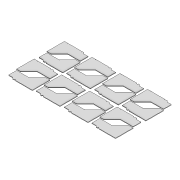
# Autodesk Inventor part: Contour_SDCard_multiple
Saved by Autodesk Inventor 2022 (Build 260153000, 153)
## iProperties
Created: 2023-04-19
Part Number: Contour_SDCard_multiple
Material: Generisch
Document SubType Name: Modeling
Designer: diederichbenedict
Density: 1 g/cm^3
Appearance: Vorgabe
Author: diederichbenedict
Autodesk Inventor part; units mm, degrees
(part 1 of 2)
ref_plane "YZ Plane" through (0, 0, 0) normal (1, 0, 0) x (0, 1, 0)
ref_plane "XZ Plane" through (0, 0, 0) normal (0, 1, 0) x (-1, 0, 0)
ref_plane "XY Plane" through (0, 0, 0) normal (0, 0, 1) x (1, 0, 0)
sketch "Skizze1" plane through (0, 0, 0) normal (0, 1, 0) x (-1, 0, 0)
  line L0 (9.6766, 36.5124) -> (7.9266, 36.5124)
  line L1 (34.6032, 1.527) -> (34.6032, 10.9706)
  line L2 (101.255, 38.0416) -> (101.255, 47.4852)
  line L3 (24.9386, 68.4228) -> (29.9386, 68.4228)
  line L4 (39.5032, 38.027) -> (34.5032, 38.027)
  line L5 (119.867, 33.452) -> (120.617, 32.702)
  line L6 (124.767, 68.452) -> (129.767, 68.452)
  line L7 (106.355, 1.5416) -> (101.355, 1.5416)
  line L8 (31.3402, 36.5124) -> (31.3402, 57.5178)
  line L9 (4.9526, 48.9174) -> (15.011, 58.9758)
  line L10 (104.781, 48.9466) -> (114.839, 59.005)
  line L11 (109.505, 36.5416) -> (107.755, 36.5416)
  line L12 (15.111, 22.4758) -> (30.0386, 22.4758)
  line L13 (77.5282, 0.777) -> (76.5282, 0.777)
  line L14 (54.7652, 69.1874) -> (54.7652, 69.9374)
  line L15 (121.517, 69.202) -> (121.517, 69.952)
  line L16 (131.168, 57.547) -> (126.241, 57.547)
  line L17 (53.0152, 69.9374) -> (53.7652, 69.1874)
  line L18 (64.5168, 21.0324) -> (59.5892, 21.0324)
  line L19 (39.6032, 1.527) -> (34.6032, 1.527)
  line L20 (78.1782, 36.527) -> (77.4282, 37.277)
  line L21 (87.5402, 32.6874) -> (88.5402, 32.6874)
  line L22 (31.3402, 57.5178) -> (26.4126, 57.5178)
  line L23 (44.5032, 36.527) -> (43.7532, 37.277)
  line L24 (53.7652, 69.1874) -> (54.7652, 69.1874)
  line L25 (126.241, 57.547) -> (116.182, 47.4886)
  line L26 (116.282, 10.9886) -> (101.355, 10.9886)
  line L27 (90.1902, 69.9374) -> (91.6902, 68.4374)
  line L28 (101.355, 1.5416) -> (101.355, 10.9852)
  line L29 (58.0152, 68.4374) -> (63.0152, 68.4374)
  line L30 (78.2782, 0.027) -> (98.1918, 0.027)
  line L31 (71.7042, 48.932) -> (81.7626, 58.9904)
  line L32 (121.617, 32.702) -> (121.617, 33.452)
  line L33 (49.5308, 10.974) -> (34.6032, 10.974)
  line L34 (88.5402, 33.4374) -> (90.2902, 33.4374)
  line L35 (31.4402, 21.0178) -> (26.5126, 21.0178)
  line L36 (90.2902, 33.4374) -> (91.7902, 31.9374)
  line L37 (111.355, 0.0416) -> (110.605, 0.7916)
  line L38 (76.4282, 37.277) -> (76.4282, 36.527)
  line L39 (9.6766, 37.2624) -> (9.6766, 36.5124)
  line L40 (86.6902, 69.9374) -> (66.7766, 69.9374)
  line L41 (111.255, 36.5416) -> (110.505, 37.2916)
  line L42 (5.0526, 12.4174) -> (15.111, 22.4758)
  line L43 (6.5266, 1.5124) -> (1.5266, 1.5124)
  line L44 (44.6032, 0.027) -> (64.5168, 0.027)
  line L45 (110.505, 37.2916) -> (109.505, 37.2916)
  line L46 (120.517, 69.202) -> (121.517, 69.202)
  line L47 (87.4402, 69.1874) -> (88.4402, 69.1874)
  line L48 (16.4542, 10.9594) -> (1.5266, 10.9594)
  line L49 (41.1032, 0.027) -> (39.6032, 1.527)
  line L50 (74.7782, 0.027) -> (73.2782, 1.527)
  line L51 (54.7652, 69.9374) -> (56.5152, 69.9374)
  line L52 (54.8652, 32.6874) -> (54.8652, 33.4374)
  line L53 (98.1918, 21.0324) -> (93.2642, 21.0324)
  line L54 (98.0918, 36.527) -> (98.0918, 57.5324)
  line L55 (129.767, 68.452) -> (129.767, 59.0084)
  line L56 (6.4266, 38.0124) -> (1.4266, 38.0124)
  line L57 (15.011, 58.9758) -> (29.9386, 58.9758)
  line L58 (1.5266, 1.5124) -> (1.5266, 10.956)
  line L59 (64.5168, 0.027) -> (64.5168, 21.0324)
  line L60 (0.025, 69.9228) -> (0.025, 48.9174)
  line L61 (21.7886, 33.4228) -> (23.5386, 33.4228)
  line L62 (64.4168, 36.527) -> (64.4168, 57.5324)
  line L63 (126.341, 21.047) -> (116.282, 10.9886)
  line L64 (66.8766, 12.432) -> (71.8042, 12.432)
  line L65 (30.0386, 31.9228) -> (30.0386, 22.4792)
  line L66 (119.767, 69.952) -> (120.517, 69.202)
  line L67 (114.939, 22.505) -> (129.867, 22.505)
  line L68 (68.1782, 38.027) -> (68.1782, 47.4706)
  line L69 (11.4266, 36.5124) -> (10.6766, 37.2624)
  line L70 (9.7766, 0.0124) -> (8.0266, 0.0124)
  line L71 (114.839, 59.005) -> (129.767, 59.005)
  line L72 (99.9532, 33.452) -> (99.9532, 12.4466)
  line L73 (11.5266, 0.0124) -> (31.4402, 0.0124)
  line L74 (71.8042, 12.432) -> (81.8626, 22.4904)
  line L75 (91.7902, 31.9374) -> (96.7902, 31.9374)
  line L76 (29.9386, 68.4228) -> (29.9386, 58.9792)
  line L77 (99.8532, 69.952) -> (99.8532, 48.9466)
  line L78 (119.767, 69.952) -> (99.8532, 69.952)
  line L79 (31.4402, 0.0124) -> (31.4402, 21.0178)
  line L80 (93.2642, 21.0324) -> (83.2058, 10.974)
  line L81 (91.6902, 68.4374) -> (96.6902, 68.4374)
  line L82 (23.4386, 69.9228) -> (24.9386, 68.4228)
  line L83 (25.0386, 31.9228) -> (30.0386, 31.9228)
  line L84 (42.7532, 37.277) -> (42.7532, 36.527)
  line L85 (8.0266, 0.0124) -> (6.5266, 1.5124)
  line L86 (66.8766, 33.4374) -> (66.8766, 12.432)
  line L87 (76.5282, 0.027) -> (74.7782, 0.027)
  line L88 (42.7532, 36.527) -> (41.0032, 36.527)
  line L89 (26.5126, 21.0178) -> (16.4542, 10.9594)
  line L90 (96.6902, 68.4374) -> (96.6902, 58.9938)
  line L91 (59.4892, 57.5324) -> (49.4308, 47.474)
  line L92 (49.4308, 47.474) -> (34.5032, 47.474)
  line L93 (20.0386, 33.4228) -> (20.7886, 32.6728)
  line L94 (26.4126, 57.5178) -> (16.3542, 47.4594)
  line L95 (109.505, 37.2916) -> (109.505, 36.5416)
  line L96 (20.6886, 69.1728) -> (21.6886, 69.1728)
  line L97 (120.617, 32.702) -> (121.617, 32.702)
  line L98 (107.755, 36.5416) -> (106.255, 38.0416)
  line L99 (123.267, 69.952) -> (124.767, 68.452)
  line L100 (86.6902, 69.9374) -> (87.4402, 69.1874)
  line L101 (48.1876, 22.4904) -> (63.1152, 22.4904)
  line L102 (21.6886, 69.9228) -> (23.4386, 69.9228)
  line L103 (56.6152, 33.4374) -> (58.1152, 31.9374)
  line L104 (1.4266, 38.0124) -> (1.4266, 47.456)
  line L105 (53.1152, 33.4374) -> (53.8652, 32.6874)
  line L106 (83.2058, 10.974) -> (68.2782, 10.974)
  line L107 (129.867, 31.952) -> (129.867, 22.5084)
  line L108 (93.1642, 57.5324) -> (83.1058, 47.474)
  line L109 (11.4266, 36.5124) -> (31.3402, 36.5124)
  line L110 (53.1152, 33.4374) -> (33.2016, 33.4374)
  line L111 (23.5386, 33.4228) -> (25.0386, 31.9228)
  line L112 (81.8626, 22.4904) -> (96.7902, 22.4904)
  line L113 (33.2016, 33.4374) -> (33.2016, 12.432)
  line L114 (42.8532, 0.777) -> (42.8532, 0.027)
  line L115 (73.2782, 1.527) -> (68.2782, 1.527)
  line L116 (20.7886, 32.6728) -> (21.7886, 32.6728)
  line L117 (73.1782, 38.027) -> (68.1782, 38.027)
  line L118 (11.5266, 0.0124) -> (10.7766, 0.7624)
  line L119 (86.7902, 33.4374) -> (87.5402, 32.6874)
  line L120 (16.3542, 47.4594) -> (1.4266, 47.4594)
  line L121 (86.7902, 33.4374) -> (66.8766, 33.4374)
  line L122 (44.6032, 0.027) -> (43.8532, 0.777)
  line L123 (43.8532, 0.777) -> (42.8532, 0.777)
  line L124 (38.0292, 48.932) -> (48.0876, 58.9904)
  line L125 (96.7902, 31.9374) -> (96.7902, 22.4938)
  line L126 (21.6886, 69.1728) -> (21.6886, 69.9228)
  line L127 (104.881, 12.4466) -> (114.939, 22.505)
  line L128 (131.268, 0.0416) -> (131.268, 21.047)
  line L129 (131.268, 21.047) -> (126.341, 21.047)
  line L130 (98.1918, 0.027) -> (98.1918, 21.0324)
  line L131 (88.4402, 69.9374) -> (90.1902, 69.9374)
  line L132 (38.1292, 12.432) -> (48.1876, 22.4904)
  line L133 (88.4402, 69.1874) -> (88.4402, 69.9374)
  line L134 (124.867, 31.952) -> (129.867, 31.952)
  line L135 (33.1016, 69.9374) -> (33.1016, 48.932)
  line L136 (10.7766, 0.7624) -> (9.7766, 0.7624)
  line L137 (43.7532, 37.277) -> (42.7532, 37.277)
  line L138 (10.6766, 37.2624) -> (9.6766, 37.2624)
  line L139 (121.517, 69.952) -> (123.267, 69.952)
  line L140 (33.1016, 48.932) -> (38.0292, 48.932)
  line L141 (81.7626, 58.9904) -> (96.6902, 58.9904)
  line L142 (76.4282, 36.527) -> (74.6782, 36.527)
  line L143 (119.867, 33.452) -> (99.9532, 33.452)
  line L144 (99.9532, 12.4466) -> (104.881, 12.4466)
  line L145 (64.4168, 57.5324) -> (59.4892, 57.5324)
  line L146 (66.7766, 48.932) -> (71.7042, 48.932)
  line L147 (110.605, 0.7916) -> (109.605, 0.7916)
  line L148 (33.2016, 12.432) -> (38.1292, 12.432)
  line L149 (78.1782, 36.527) -> (98.0918, 36.527)
  line L150 (56.5152, 69.9374) -> (58.0152, 68.4374)
  line L151 (34.5032, 38.027) -> (34.5032, 47.4706)
  line L152 (48.0876, 58.9904) -> (63.0152, 58.9904)
  line L153 (7.9266, 36.5124) -> (6.4266, 38.0124)
  line L154 (121.617, 33.452) -> (123.367, 33.452)
  line L155 (63.0152, 68.4374) -> (63.0152, 58.9938)
  line L156 (0.025, 48.9174) -> (4.9526, 48.9174)
  line L157 (99.8532, 48.9466) -> (104.781, 48.9466)
  line L158 (74.6782, 36.527) -> (73.1782, 38.027)
  line L159 (109.605, 0.0416) -> (107.855, 0.0416)
  line L160 (98.0918, 57.5324) -> (93.1642, 57.5324)
  line L161 (116.182, 47.4886) -> (101.255, 47.4886)
  line L162 (42.8532, 0.027) -> (41.1032, 0.027)
  line L163 (53.8652, 32.6874) -> (54.8652, 32.6874)
  line L164 (123.367, 33.452) -> (124.867, 31.952)
  line L165 (63.1152, 31.9374) -> (63.1152, 22.4938)
  line L166 (44.5032, 36.527) -> (64.4168, 36.527)
  line L167 (0.125, 33.4228) -> (0.125, 12.4174)
  line L168 (76.5282, 0.777) -> (76.5282, 0.027)
  line L169 (111.255, 36.5416) -> (131.168, 36.5416)
  line L170 (19.9386, 69.9228) -> (20.6886, 69.1728)
  line L171 (106.255, 38.0416) -> (101.255, 38.0416)
  line L172 (66.7766, 69.9374) -> (66.7766, 48.932)
  line L173 (109.605, 0.7916) -> (109.605, 0.0416)
  line L174 (21.7886, 32.6728) -> (21.7886, 33.4228)
  line L175 (20.0386, 33.4228) -> (0.125, 33.4228)
  line L176 (107.855, 0.0416) -> (106.355, 1.5416)
  line L177 (131.168, 36.5416) -> (131.168, 57.547)
  line L178 (53.0152, 69.9374) -> (33.1016, 69.9374)
  line L179 (59.5892, 21.0324) -> (49.5308, 10.974)
  line L180 (78.2782, 0.027) -> (77.5282, 0.777)
  line L181 (19.9386, 69.9228) -> (0.025, 69.9228)
  line L182 (58.1152, 31.9374) -> (63.1152, 31.9374)
  line L183 (41.0032, 36.527) -> (39.5032, 38.027)
  line L184 (88.5402, 32.6874) -> (88.5402, 33.4374)
  line L185 (54.8652, 33.4374) -> (56.6152, 33.4374)
  line L186 (83.1058, 47.474) -> (68.1782, 47.474)
  line L187 (9.7766, 0.7624) -> (9.7766, 0.0124)
  line L188 (111.355, 0.0416) -> (131.268, 0.0416)
  line L189 (68.2782, 1.527) -> (68.2782, 10.9706)
  line L190 (0.125, 12.4174) -> (5.0526, 12.4174)
  line L191 (77.4282, 37.277) -> (76.4282, 37.277)
  line L192 (93.9699, 35.8046) -> (93.6365, 36.2808)
  line L193 (93.3984, 35.8046) -> (93.3984, 36.8046)
  line L194 (93.3984, 36.8046) -> (93.7794, 36.8046)
  line L195 (93.7794, 36.8046) -> (93.8746, 36.757)
  line L196 (93.8746, 36.757) -> (93.9222, 36.7094)
  line L197 (93.9222, 36.7094) -> (93.9699, 36.6141)
  line L198 (93.9699, 36.6141) -> (93.9699, 36.4713)
  line L199 (93.9699, 36.4713) -> (93.9222, 36.376)
  line L200 (93.9222, 36.376) -> (93.8746, 36.3284)
  line L201 (93.8746, 36.3284) -> (93.7794, 36.2808)
  line L202 (93.7794, 36.2808) -> (93.3984, 36.2808)
  line L203 (94.3984, 36.3284) -> (94.7318, 36.3284)
  line L204 (94.8746, 35.8046) -> (94.3984, 35.8046)
  line L205 (94.3984, 35.8046) -> (94.3984, 36.8046)
  line L206 (94.3984, 36.8046) -> (94.8746, 36.8046)
  line L207 (95.6365, 36.3284) -> (95.3032, 36.3284)
  line L208 (95.3032, 35.8046) -> (95.3032, 36.8046)
  line L209 (95.3032, 36.8046) -> (95.7794, 36.8046)
  line L210 (96.3032, 36.8046) -> (96.3032, 36.5665)
  line L211 (96.0651, 36.6618) -> (96.3032, 36.5665)
  line L212 (96.3032, 36.5665) -> (96.5413, 36.6618)
  line L213 (96.1603, 36.376) -> (96.3032, 36.5665)
  line L214 (96.3032, 36.5665) -> (96.4461, 36.376)
  line L215 (97.0651, 36.8046) -> (97.0651, 36.5665)
  line L216 (96.827, 36.6618) -> (97.0651, 36.5665)
  line L217 (97.0651, 36.5665) -> (97.3032, 36.6618)
  line L218 (96.9222, 36.376) -> (97.0651, 36.5665)
  line L219 (97.0651, 36.5665) -> (97.208, 36.376)
  line L220 (34.5569, 69.925) -> (34.2235, 70.4012)
  line L221 (33.9854, 69.925) -> (33.9854, 70.925)
  line L222 (33.9854, 70.925) -> (34.3664, 70.925)
  line L223 (34.3664, 70.925) -> (34.4616, 70.8774)
  line L224 (34.4616, 70.8774) -> (34.5092, 70.8298)
  line L225 (34.5092, 70.8298) -> (34.5569, 70.7345)
  line L226 (34.5569, 70.7345) -> (34.5569, 70.5917)
  line L227 (34.5569, 70.5917) -> (34.5092, 70.4964)
  line L228 (34.5092, 70.4964) -> (34.4616, 70.4488)
  line L229 (34.4616, 70.4488) -> (34.3664, 70.4012)
  line L230 (34.3664, 70.4012) -> (33.9854, 70.4012)
  line L231 (34.9854, 70.4488) -> (35.3188, 70.4488)
  line L232 (35.4616, 69.925) -> (34.9854, 69.925)
  line L233 (34.9854, 69.925) -> (34.9854, 70.925)
  line L234 (34.9854, 70.925) -> (35.4616, 70.925)
  line L235 (36.2235, 70.4488) -> (35.8902, 70.4488)
  line L236 (35.8902, 69.925) -> (35.8902, 70.925)
  line L237 (35.8902, 70.925) -> (36.3664, 70.925)
  line L238 (36.8902, 70.925) -> (36.8902, 70.6869)
  line L239 (36.6521, 70.7822) -> (36.8902, 70.6869)
  line L240 (36.8902, 70.6869) -> (37.1283, 70.7822)
  line L241 (36.7473, 70.4964) -> (36.8902, 70.6869)
  line L242 (36.8902, 70.6869) -> (37.0331, 70.4964)
  line L243 (37.6521, 70.925) -> (37.6521, 70.6869)
  line L244 (37.414, 70.7822) -> (37.6521, 70.6869)
  line L245 (37.6521, 70.6869) -> (37.8902, 70.7822)
  line L246 (37.5092, 70.4964) -> (37.6521, 70.6869)
  line L247 (37.6521, 70.6869) -> (37.795, 70.4964)
  line L248 (68.3319, 33.425) -> (67.9985, 33.9012)
  line L249 (67.7604, 33.425) -> (67.7604, 34.425)
  line L250 (67.7604, 34.425) -> (68.1414, 34.425)
  line L251 (68.1414, 34.425) -> (68.2366, 34.3774)
  line L252 (68.2366, 34.3774) -> (68.2842, 34.3298)
  line L253 (68.2842, 34.3298) -> (68.3319, 34.2345)
  line L254 (68.3319, 34.2345) -> (68.3319, 34.0917)
  line L255 (68.3319, 34.0917) -> (68.2842, 33.9964)
  line L256 (68.2842, 33.9964) -> (68.2366, 33.9488)
  line L257 (68.2366, 33.9488) -> (68.1414, 33.9012)
  line L258 (68.1414, 33.9012) -> (67.7604, 33.9012)
  line L259 (68.7604, 33.9488) -> (69.0938, 33.9488)
  line L260 (69.2366, 33.425) -> (68.7604, 33.425)
  line L261 (68.7604, 33.425) -> (68.7604, 34.425)
  line L262 (68.7604, 34.425) -> (69.2366, 34.425)
  line L263 (69.9985, 33.9488) -> (69.6652, 33.9488)
  line L264 (69.6652, 33.425) -> (69.6652, 34.425)
  line L265 (69.6652, 34.425) -> (70.1414, 34.425)
  line L266 (70.6652, 34.425) -> (70.6652, 34.1869)
  line L267 (70.4271, 34.2822) -> (70.6652, 34.1869)
  line L268 (70.6652, 34.1869) -> (70.9033, 34.2822)
  line L269 (70.5223, 33.9964) -> (70.6652, 34.1869)
  line L270 (70.6652, 34.1869) -> (70.8081, 33.9964)
  line L271 (71.4271, 34.425) -> (71.4271, 34.1869)
  line L272 (71.189, 34.2822) -> (71.4271, 34.1869)
  line L273 (71.4271, 34.1869) -> (71.6652, 34.2822)
  line L274 (71.2842, 33.9964) -> (71.4271, 34.1869)
  line L275 (71.4271, 34.1869) -> (71.57, 33.9964)
  line L276 (101.308, 69.9396) -> (100.975, 70.4158)
  line L277 (100.737, 69.9396) -> (100.737, 70.9396)
  line L278 (100.737, 70.9396) -> (101.118, 70.9396)
  line L279 (101.118, 70.9396) -> (101.213, 70.892)
  line L280 (101.213, 70.892) -> (101.261, 70.8444)
  line L281 (101.261, 70.8444) -> (101.308, 70.7491)
  line L282 (101.308, 70.7491) -> (101.308, 70.6063)
  line L283 (101.308, 70.6063) -> (101.261, 70.511)
  line L284 (101.261, 70.511) -> (101.213, 70.4634)
  line L285 (101.213, 70.4634) -> (101.118, 70.4158)
  line L286 (101.118, 70.4158) -> (100.737, 70.4158)
  line L287 (101.737, 70.4634) -> (102.07, 70.4634)
  line L288 (102.213, 69.9396) -> (101.737, 69.9396)
  line L289 (101.737, 69.9396) -> (101.737, 70.9396)
  line L290 (101.737, 70.9396) -> (102.213, 70.9396)
  line L291 (102.975, 70.4634) -> (102.642, 70.4634)
  line L292 (102.642, 69.9396) -> (102.642, 70.9396)
  line L293 (102.642, 70.9396) -> (103.118, 70.9396)
  line L294 (103.642, 70.9396) -> (103.642, 70.7015)
  line L295 (103.404, 70.7968) -> (103.642, 70.7015)
  line L296 (103.642, 70.7015) -> (103.88, 70.7968)
  line L297 (103.499, 70.511) -> (103.642, 70.7015)
  line L298 (103.642, 70.7015) -> (103.785, 70.511)
  line L299 (104.404, 70.9396) -> (104.404, 70.7015)
  line L300 (104.166, 70.7968) -> (104.404, 70.7015)
  line L301 (104.404, 70.7015) -> (104.642, 70.7968)
  line L302 (104.261, 70.511) -> (104.404, 70.7015)
  line L303 (104.404, 70.7015) -> (104.547, 70.511)
  line L304 (27.3183, -0.71) -> (26.9849, -0.2338)
  line L305 (26.7468, -0.71) -> (26.7468, 0.29)
  line L306 (26.7468, 0.29) -> (27.1278, 0.29)
  line L307 (27.1278, 0.29) -> (27.223, 0.2424)
  line L308 (27.223, 0.2424) -> (27.2706, 0.1948)
  line L309 (27.2706, 0.1948) -> (27.3183, 0.0995)
  line L310 (27.3183, 0.0995) -> (27.3183, -0.0433)
  line L311 (27.3183, -0.0433) -> (27.2706, -0.1386)
  line L312 (27.2706, -0.1386) -> (27.223, -0.1862)
  line L313 (27.223, -0.1862) -> (27.1278, -0.2338)
  line L314 (27.1278, -0.2338) -> (26.7468, -0.2338)
  line L315 (27.7468, -0.1862) -> (28.0802, -0.1862)
  line L316 (28.223, -0.71) -> (27.7468, -0.71)
  line L317 (27.7468, -0.71) -> (27.7468, 0.29)
  line L318 (27.7468, 0.29) -> (28.223, 0.29)
  line L319 (28.9849, -0.1862) -> (28.6516, -0.1862)
  line L320 (28.6516, -0.71) -> (28.6516, 0.29)
  line L321 (28.6516, 0.29) -> (29.1278, 0.29)
  line L322 (29.6516, 0.29) -> (29.6516, 0.0519)
  line L323 (29.4135, 0.1472) -> (29.6516, 0.0519)
  line L324 (29.6516, 0.0519) -> (29.8897, 0.1472)
  line L325 (29.5087, -0.1386) -> (29.6516, 0.0519)
  line L326 (29.6516, 0.0519) -> (29.7945, -0.1386)
  line L327 (30.4135, 0.29) -> (30.4135, 0.0519)
  line L328 (30.1754, 0.1472) -> (30.4135, 0.0519)
  line L329 (30.4135, 0.0519) -> (30.6516, 0.1472)
  line L330 (30.2706, -0.1386) -> (30.4135, 0.0519)
  line L331 (30.4135, 0.0519) -> (30.5564, -0.1386)
  line L332 (127.147, -0.6808) -> (126.813, -0.2046)
  line L333 (126.575, -0.6808) -> (126.575, 0.3192)
  line L334 (126.575, 0.3192) -> (126.956, 0.3192)
  line L335 (126.956, 0.3192) -> (127.051, 0.2716)
  line L336 (127.051, 0.2716) -> (127.099, 0.224)
  line L337 (127.099, 0.224) -> (127.147, 0.1287)
  line L338 (127.147, 0.1287) -> (127.147, -0.0141)
  line L339 (127.147, -0.0141) -> (127.099, -0.1094)
  line L340 (127.099, -0.1094) -> (127.051, -0.157)
  line L341 (127.051, -0.157) -> (126.956, -0.2046)
  line L342 (126.956, -0.2046) -> (126.575, -0.2046)
  line L343 (127.575, -0.157) -> (127.908, -0.157)
  line L344 (128.051, -0.6808) -> (127.575, -0.6808)
  line L345 (127.575, -0.6808) -> (127.575, 0.3192)
  line L346 (127.575, 0.3192) -> (128.051, 0.3192)
  line L347 (128.813, -0.157) -> (128.48, -0.157)
  line L348 (128.48, -0.6808) -> (128.48, 0.3192)
  line L349 (128.48, 0.3192) -> (128.956, 0.3192)
  line L350 (129.48, 0.3192) -> (129.48, 0.0811)
  line L351 (129.242, 0.1764) -> (129.48, 0.0811)
  line L352 (129.48, 0.0811) -> (129.718, 0.1764)
  line L353 (129.337, -0.1094) -> (129.48, 0.0811)
  line L354 (129.48, 0.0811) -> (129.623, -0.1094)
  line L355 (130.242, 0.3192) -> (130.242, 0.0811)
  line L356 (130.004, 0.1764) -> (130.242, 0.0811)
  line L357 (130.242, 0.0811) -> (130.48, 0.1764)
  line L358 (130.099, -0.1094) -> (130.242, 0.0811)
  line L359 (130.242, 0.0811) -> (130.385, -0.1094)
  line L360 (1.5803, 33.4104) -> (1.2469, 33.8866)
  line L361 (1.0088, 33.4104) -> (1.0088, 34.4104)
  line L362 (1.0088, 34.4104) -> (1.3898, 34.4104)
  line L363 (1.3898, 34.4104) -> (1.485, 34.3628)
  line L364 (1.485, 34.3628) -> (1.5326, 34.3152)
  line L365 (1.5326, 34.3152) -> (1.5803, 34.2199)
  line L366 (1.5803, 34.2199) -> (1.5803, 34.0771)
  line L367 (1.5803, 34.0771) -> (1.5326, 33.9818)
  line L368 (1.5326, 33.9818) -> (1.485, 33.9342)
  line L369 (1.485, 33.9342) -> (1.3898, 33.8866)
  line L370 (1.3898, 33.8866) -> (1.0088, 33.8866)
  line L371 (2.0088, 33.9342) -> (2.3422, 33.9342)
  line L372 (2.485, 33.4104) -> (2.0088, 33.4104)
  line L373 (2.0088, 33.4104) -> (2.0088, 34.4104)
  line L374 (2.0088, 34.4104) -> (2.485, 34.4104)
  line L375 (3.2469, 33.9342) -> (2.9136, 33.9342)
  line L376 (2.9136, 33.4104) -> (2.9136, 34.4104)
  line L377 (2.9136, 34.4104) -> (3.3898, 34.4104)
  line L378 (3.9136, 34.4104) -> (3.9136, 34.1723)
  line L379 (3.6755, 34.2676) -> (3.9136, 34.1723)
  line L380 (3.9136, 34.1723) -> (4.1517, 34.2676)
  line L381 (3.7707, 33.9818) -> (3.9136, 34.1723)
  line L382 (3.9136, 34.1723) -> (4.0565, 33.9818)
  line L383 (4.6755, 34.4104) -> (4.6755, 34.1723)
  line L384 (4.4374, 34.2676) -> (4.6755, 34.1723)
  line L385 (4.6755, 34.1723) -> (4.9136, 34.2676)
  line L386 (4.5326, 33.9818) -> (4.6755, 34.1723)
  line L387 (4.6755, 34.1723) -> (4.8184, 33.9818)
  line L388 (60.2949, 35.8046) -> (59.9615, 36.2808)
  line L389 (59.7234, 35.8046) -> (59.7234, 36.8046)
  line L390 (59.7234, 36.8046) -> (60.1044, 36.8046)
  line L391 (60.1044, 36.8046) -> (60.1996, 36.757)
  line L392 (60.1996, 36.757) -> (60.2472, 36.7094)
  line L393 (60.2472, 36.7094) -> (60.2949, 36.6141)
  line L394 (60.2949, 36.6141) -> (60.2949, 36.4713)
  line L395 (60.2949, 36.4713) -> (60.2472, 36.376)
  line L396 (60.2472, 36.376) -> (60.1996, 36.3284)
  line L397 (60.1996, 36.3284) -> (60.1044, 36.2808)
  line L398 (60.1044, 36.2808) -> (59.7234, 36.2808)
  line L399 (60.7234, 36.3284) -> (61.0568, 36.3284)
  line L400 (61.1996, 35.8046) -> (60.7234, 35.8046)
  line L401 (60.7234, 35.8046) -> (60.7234, 36.8046)
  line L402 (60.7234, 36.8046) -> (61.1996, 36.8046)
  line L403 (61.9615, 36.3284) -> (61.6282, 36.3284)
  line L404 (61.6282, 35.8046) -> (61.6282, 36.8046)
  line L405 (61.6282, 36.8046) -> (62.1044, 36.8046)
  line L406 (62.6282, 36.8046) -> (62.6282, 36.5665)
  line L407 (62.3901, 36.6618) -> (62.6282, 36.5665)
  line L408 (62.6282, 36.5665) -> (62.8663, 36.6618)
  line L409 (62.4853, 36.376) -> (62.6282, 36.5665)
  line L410 (62.6282, 36.5665) -> (62.7711, 36.376)
  line L411 (63.3901, 36.8046) -> (63.3901, 36.5665)
  line L412 (63.152, 36.6618) -> (63.3901, 36.5665)
  line L413 (63.3901, 36.5665) -> (63.6282, 36.6618)
  line L414 (63.2472, 36.376) -> (63.3901, 36.5665)
  line L415 (63.3901, 36.5665) -> (63.533, 36.376)
  line L416 (94.0699, -0.6954) -> (93.7365, -0.2192)
  line L417 (93.4984, -0.6954) -> (93.4984, 0.3046)
  line L418 (93.4984, 0.3046) -> (93.8794, 0.3046)
  line L419 (93.8794, 0.3046) -> (93.9746, 0.257)
  line L420 (93.9746, 0.257) -> (94.0222, 0.2094)
  line L421 (94.0222, 0.2094) -> (94.0699, 0.1141)
  line L422 (94.0699, 0.1141) -> (94.0699, -0.0287)
  line L423 (94.0699, -0.0287) -> (94.0222, -0.124)
  line L424 (94.0222, -0.124) -> (93.9746, -0.1716)
  line L425 (93.9746, -0.1716) -> (93.8794, -0.2192)
  line L426 (93.8794, -0.2192) -> (93.4984, -0.2192)
  line L427 (94.4984, -0.1716) -> (94.8318, -0.1716)
  line L428 (94.9746, -0.6954) -> (94.4984, -0.6954)
  line L429 (94.4984, -0.6954) -> (94.4984, 0.3046)
  line L430 (94.4984, 0.3046) -> (94.9746, 0.3046)
  line L431 (95.7365, -0.1716) -> (95.4032, -0.1716)
  line L432 (95.4032, -0.6954) -> (95.4032, 0.3046)
  line L433 (95.4032, 0.3046) -> (95.8794, 0.3046)
  line L434 (96.4032, 0.3046) -> (96.4032, 0.0665)
  line L435 (96.1651, 0.1618) -> (96.4032, 0.0665)
  line L436 (96.4032, 0.0665) -> (96.6413, 0.1618)
  line L437 (96.2603, -0.124) -> (96.4032, 0.0665)
  line L438 (96.4032, 0.0665) -> (96.5461, -0.124)
  line L439 (97.1651, 0.3046) -> (97.1651, 0.0665)
  line L440 (96.927, 0.1618) -> (97.1651, 0.0665)
  line L441 (97.1651, 0.0665) -> (97.4032, 0.1618)
  line L442 (97.0222, -0.124) -> (97.1651, 0.0665)
  line L443 (97.1651, 0.0665) -> (97.308, -0.124)
  line L444 (68.2319, 69.925) -> (67.8985, 70.4012)
  line L445 (67.6604, 69.925) -> (67.6604, 70.925)
  line L446 (67.6604, 70.925) -> (68.0414, 70.925)
  line L447 (68.0414, 70.925) -> (68.1366, 70.8774)
  line L448 (68.1366, 70.8774) -> (68.1842, 70.8298)
  line L449 (68.1842, 70.8298) -> (68.2319, 70.7345)
  line L450 (68.2319, 70.7345) -> (68.2319, 70.5917)
  line L451 (68.2319, 70.5917) -> (68.1842, 70.4964)
  line L452 (68.1842, 70.4964) -> (68.1366, 70.4488)
  line L453 (68.1366, 70.4488) -> (68.0414, 70.4012)
  line L454 (68.0414, 70.4012) -> (67.6604, 70.4012)
  line L455 (68.6604, 70.4488) -> (68.9938, 70.4488)
  line L456 (69.1366, 69.925) -> (68.6604, 69.925)
  line L457 (68.6604, 69.925) -> (68.6604, 70.925)
  line L458 (68.6604, 70.925) -> (69.1366, 70.925)
  line L459 (69.8985, 70.4488) -> (69.5652, 70.4488)
  line L460 (69.5652, 69.925) -> (69.5652, 70.925)
  line L461 (69.5652, 70.925) -> (70.0414, 70.925)
  line L462 (70.5652, 70.925) -> (70.5652, 70.6869)
  line L463 (70.3271, 70.7822) -> (70.5652, 70.6869)
  line L464 (70.5652, 70.6869) -> (70.8033, 70.7822)
  line L465 (70.4223, 70.4964) -> (70.5652, 70.6869)
  line L466 (70.5652, 70.6869) -> (70.7081, 70.4964)
  line L467 (71.3271, 70.925) -> (71.3271, 70.6869)
  line L468 (71.089, 70.7822) -> (71.3271, 70.6869)
  line L469 (71.3271, 70.6869) -> (71.5652, 70.7822)
  line L470 (71.1842, 70.4964) -> (71.3271, 70.6869)
  line L471 (71.3271, 70.6869) -> (71.47, 70.4964)
  line L472 (1.4803, 69.9104) -> (1.1469, 70.3866)
  line L473 (0.9088, 69.9104) -> (0.9088, 70.9104)
  line L474 (0.9088, 70.9104) -> (1.2898, 70.9104)
  line L475 (1.2898, 70.9104) -> (1.385, 70.8628)
  line L476 (1.385, 70.8628) -> (1.4326, 70.8152)
  line L477 (1.4326, 70.8152) -> (1.4803, 70.7199)
  line L478 (1.4803, 70.7199) -> (1.4803, 70.5771)
  line L479 (1.4803, 70.5771) -> (1.4326, 70.4818)
  line L480 (1.4326, 70.4818) -> (1.385, 70.4342)
  line L481 (1.385, 70.4342) -> (1.2898, 70.3866)
  line L482 (1.2898, 70.3866) -> (0.9088, 70.3866)
  line L483 (1.9088, 70.4342) -> (2.2422, 70.4342)
  line L484 (2.385, 69.9104) -> (1.9088, 69.9104)
  line L485 (1.9088, 69.9104) -> (1.9088, 70.9104)
  line L486 (1.9088, 70.9104) -> (2.385, 70.9104)
  line L487 (3.1469, 70.4342) -> (2.8136, 70.4342)
  line L488 (2.8136, 69.9104) -> (2.8136, 70.9104)
  line L489 (2.8136, 70.9104) -> (3.2898, 70.9104)
  line L490 (3.8136, 70.9104) -> (3.8136, 70.6723)
  line L491 (3.5755, 70.7676) -> (3.8136, 70.6723)
  line L492 (3.8136, 70.6723) -> (4.0517, 70.7676)
  line L493 (3.6707, 70.4818) -> (3.8136, 70.6723)
  line L494 (3.8136, 70.6723) -> (3.9565, 70.4818)
  line L495 (4.5755, 70.9104) -> (4.5755, 70.6723)
  line L496 (4.3374, 70.7676) -> (4.5755, 70.6723)
  line L497 (4.5755, 70.6723) -> (4.8136, 70.7676)
  line L498 (4.4326, 70.4818) -> (4.5755, 70.6723)
  line L499 (4.5755, 70.6723) -> (4.7184, 70.4818)
  line L500 (27.2183, 35.79) -> (26.8849, 36.2662)
  line L501 (26.6468, 35.79) -> (26.6468, 36.79)
  line L502 (26.6468, 36.79) -> (27.0278, 36.79)
  line L503 (27.0278, 36.79) -> (27.123, 36.7424)
  line L504 (27.123, 36.7424) -> (27.1706, 36.6948)
  line L505 (27.1706, 36.6948) -> (27.2183, 36.5995)
  line L506 (27.2183, 36.5995) -> (27.2183, 36.4567)
  line L507 (27.2183, 36.4567) -> (27.1706, 36.3614)
  line L508 (27.1706, 36.3614) -> (27.123, 36.3138)
  line L509 (27.123, 36.3138) -> (27.0278, 36.2662)
  line L510 (27.0278, 36.2662) -> (26.6468, 36.2662)
  line L511 (27.6468, 36.3138) -> (27.9802, 36.3138)
  line L512 (28.123, 35.79) -> (27.6468, 35.79)
  line L513 (27.6468, 35.79) -> (27.6468, 36.79)
  line L514 (27.6468, 36.79) -> (28.123, 36.79)
  line L515 (28.8849, 36.3138) -> (28.5516, 36.3138)
  line L516 (28.5516, 35.79) -> (28.5516, 36.79)
  line L517 (28.5516, 36.79) -> (29.0278, 36.79)
  line L518 (29.5516, 36.79) -> (29.5516, 36.5519)
  line L519 (29.3135, 36.6472) -> (29.5516, 36.5519)
  line L520 (29.5516, 36.5519) -> (29.7897, 36.6472)
  line L521 (29.4087, 36.3614) -> (29.5516, 36.5519)
  line L522 (29.5516, 36.5519) -> (29.6945, 36.3614)
  line L523 (30.3135, 36.79) -> (30.3135, 36.5519)
  line L524 (30.0754, 36.6472) -> (30.3135, 36.5519)
  line L525 (30.3135, 36.5519) -> (30.5516, 36.6472)
  line L526 (30.1706, 36.3614) -> (30.3135, 36.5519)
  line L527 (30.3135, 36.5519) -> (30.4564, 36.3614)
  line L528 (34.6569, 33.425) -> (34.3235, 33.9012)
  line L529 (34.0854, 33.425) -> (34.0854, 34.425)
  line L530 (34.0854, 34.425) -> (34.4664, 34.425)
  line L531 (34.4664, 34.425) -> (34.5616, 34.3774)
  line L532 (34.5616, 34.3774) -> (34.6092, 34.3298)
  line L533 (34.6092, 34.3298) -> (34.6569, 34.2345)
  line L534 (34.6569, 34.2345) -> (34.6569, 34.0917)
  line L535 (34.6569, 34.0917) -> (34.6092, 33.9964)
  line L536 (34.6092, 33.9964) -> (34.5616, 33.9488)
  line L537 (34.5616, 33.9488) -> (34.4664, 33.9012)
  line L538 (34.4664, 33.9012) -> (34.0854, 33.9012)
  line L539 (35.0854, 33.9488) -> (35.4188, 33.9488)
  line L540 (35.5616, 33.425) -> (35.0854, 33.425)
  line L541 (35.0854, 33.425) -> (35.0854, 34.425)
  line L542 (35.0854, 34.425) -> (35.5616, 34.425)
  line L543 (36.3235, 33.9488) -> (35.9902, 33.9488)
  line L544 (35.9902, 33.425) -> (35.9902, 34.425)
  line L545 (35.9902, 34.425) -> (36.4664, 34.425)
  line L546 (36.9902, 34.425) -> (36.9902, 34.1869)
  line L547 (36.7521, 34.2822) -> (36.9902, 34.1869)
  line L548 (36.9902, 34.1869) -> (37.2283, 34.2822)
  line L549 (36.8473, 33.9964) -> (36.9902, 34.1869)
  line L550 (36.9902, 34.1869) -> (37.1331, 33.9964)
  line L551 (37.7521, 34.425) -> (37.7521, 34.1869)
  line L552 (37.514, 34.2822) -> (37.7521, 34.1869)
  line L553 (37.7521, 34.1869) -> (37.9902, 34.2822)
  line L554 (37.6092, 33.9964) -> (37.7521, 34.1869)
  line L555 (37.7521, 34.1869) -> (37.895, 33.9964)
  line L556 (101.409, 33.4396) -> (101.075, 33.9158)
  line L557 (100.837, 33.4396) -> (100.837, 34.4396)
  line L558 (100.837, 34.4396) -> (101.218, 34.4396)
  line L559 (101.218, 34.4396) -> (101.313, 34.392)
  line L560 (101.313, 34.392) -> (101.361, 34.3444)
  line L561 (101.361, 34.3444) -> (101.409, 34.2491)
  line L562 (101.409, 34.2491) -> (101.409, 34.1063)
  line L563 (101.409, 34.1063) -> (101.361, 34.011)
  line L564 (101.361, 34.011) -> (101.313, 33.9634)
  line L565 (101.313, 33.9634) -> (101.218, 33.9158)
  line L566 (101.218, 33.9158) -> (100.837, 33.9158)
  line L567 (101.837, 33.9634) -> (102.17, 33.9634)
  line L568 (102.313, 33.4396) -> (101.837, 33.4396)
  line L569 (101.837, 33.4396) -> (101.837, 34.4396)
  line L570 (101.837, 34.4396) -> (102.313, 34.4396)
  line L571 (103.075, 33.9634) -> (102.742, 33.9634)
  line L572 (102.742, 33.4396) -> (102.742, 34.4396)
  line L573 (102.742, 34.4396) -> (103.218, 34.4396)
  line L574 (103.742, 34.4396) -> (103.742, 34.2015)
  line L575 (103.504, 34.2968) -> (103.742, 34.2015)
  line L576 (103.742, 34.2015) -> (103.98, 34.2968)
  line L577 (103.599, 34.011) -> (103.742, 34.2015)
  line L578 (103.742, 34.2015) -> (103.885, 34.011)
  line L579 (104.504, 34.4396) -> (104.504, 34.2015)
  line L580 (104.266, 34.2968) -> (104.504, 34.2015)
  line L581 (104.504, 34.2015) -> (104.742, 34.2968)
  line L582 (104.361, 34.011) -> (104.504, 34.2015)
  line L583 (104.504, 34.2015) -> (104.647, 34.011)
  line L584 (127.046, 35.8192) -> (126.713, 36.2954)
  line L585 (126.475, 35.8192) -> (126.475, 36.8192)
  line L586 (126.475, 36.8192) -> (126.856, 36.8192)
  line L587 (126.856, 36.8192) -> (126.951, 36.7716)
  line L588 (126.951, 36.7716) -> (126.999, 36.724)
  line L589 (126.999, 36.724) -> (127.046, 36.6287)
  line L590 (127.046, 36.6287) -> (127.046, 36.4859)
  line L591 (127.046, 36.4859) -> (126.999, 36.3906)
  line L592 (126.999, 36.3906) -> (126.951, 36.343)
  line L593 (126.951, 36.343) -> (126.856, 36.2954)
  line L594 (126.856, 36.2954) -> (126.475, 36.2954)
  line L595 (127.475, 36.343) -> (127.808, 36.343)
  line L596 (127.951, 35.8192) -> (127.475, 35.8192)
  line L597 (127.475, 35.8192) -> (127.475, 36.8192)
  line L598 (127.475, 36.8192) -> (127.951, 36.8192)
  line L599 (128.713, 36.343) -> (128.38, 36.343)
  line L600 (128.38, 35.8192) -> (128.38, 36.8192)
  line L601 (128.38, 36.8192) -> (128.856, 36.8192)
  line L602 (129.38, 36.8192) -> (129.38, 36.5811)
  line L603 (129.142, 36.6764) -> (129.38, 36.5811)
  line L604 (129.38, 36.5811) -> (129.618, 36.6764)
  line L605 (129.237, 36.3906) -> (129.38, 36.5811)
  line L606 (129.38, 36.5811) -> (129.523, 36.3906)
  line L607 (130.142, 36.8192) -> (130.142, 36.5811)
  line L608 (129.904, 36.6764) -> (130.142, 36.5811)
  line L609 (130.142, 36.5811) -> (130.38, 36.6764)
  line L610 (129.999, 36.3906) -> (130.142, 36.5811)
  line L611 (130.142, 36.5811) -> (130.285, 36.3906)
  line L612 (60.3949, -0.6954) -> (60.0615, -0.2192)
  line L613 (59.8234, -0.6954) -> (59.8234, 0.3046)
  line L614 (59.8234, 0.3046) -> (60.2044, 0.3046)
  line L615 (60.2044, 0.3046) -> (60.2996, 0.257)
  line L616 (60.2996, 0.257) -> (60.3472, 0.2094)
  line L617 (60.3472, 0.2094) -> (60.3949, 0.1141)
  line L618 (60.3949, 0.1141) -> (60.3949, -0.0287)
  line L619 (60.3949, -0.0287) -> (60.3472, -0.124)
  line L620 (60.3472, -0.124) -> (60.2996, -0.1716)
  line L621 (60.2996, -0.1716) -> (60.2044, -0.2192)
  line L622 (60.2044, -0.2192) -> (59.8234, -0.2192)
  line L623 (60.8234, -0.1716) -> (61.1568, -0.1716)
  line L624 (61.2996, -0.6954) -> (60.8234, -0.6954)
  line L625 (60.8234, -0.6954) -> (60.8234, 0.3046)
  line L626 (60.8234, 0.3046) -> (61.2996, 0.3046)
  line L627 (62.0615, -0.1716) -> (61.7282, -0.1716)
  line L628 (61.7282, -0.6954) -> (61.7282, 0.3046)
  line L629 (61.7282, 0.3046) -> (62.2044, 0.3046)
  line L630 (62.7282, 0.3046) -> (62.7282, 0.0665)
  line L631 (62.4901, 0.1618) -> (62.7282, 0.0665)
  line L632 (62.7282, 0.0665) -> (62.9663, 0.1618)
  line L633 (62.5853, -0.124) -> (62.7282, 0.0665)
  line L634 (62.7282, 0.0665) -> (62.8711, -0.124)
  line L635 (63.4901, 0.3046) -> (63.4901, 0.0665)
  line L636 (63.252, 0.1618) -> (63.4901, 0.0665)
  line L637 (63.4901, 0.0665) -> (63.7282, 0.1618)
  line L638 (63.3472, -0.124) -> (63.4901, 0.0665)
  line L639 (63.4901, 0.0665) -> (63.633, -0.124)
  line L640 (96.6332, 37.172) -> (95.3032, 37.172)
  line L641 (96.6332, 38.502) -> (96.6332, 37.172)
  line L642 (96.6332, 39.772) -> (96.6332, 57.612)
  line L643 (96.6332, 39.772) -> (93.9732, 39.772)
  line L644 (96.6332, 57.612) -> (93.9732, 57.612)
  line L645 (93.9732, 39.772) -> (93.9732, 57.612)
  line L646 (34.5602, 69.2924) -> (35.8902, 69.2924)
  line L647 (34.5602, 67.9624) -> (34.5602, 69.2924)
  line L648 (34.5602, 66.6924) -> (34.5602, 48.8524)
  line L649 (34.5602, 66.6924) -> (37.2202, 66.6924)
  line L650 (34.5602, 48.8524) -> (37.2202, 48.8524)
  line L651 (37.2202, 66.6924) -> (37.2202, 48.8524)
  line L652 (68.3352, 32.7924) -> (69.6652, 32.7924)
  line L653 (68.3352, 31.4624) -> (68.3352, 32.7924)
  line L654 (68.3352, 30.1924) -> (68.3352, 12.3524)
  line L655 (68.3352, 30.1924) -> (70.9952, 30.1924)
  line L656 (68.3352, 12.3524) -> (70.9952, 12.3524)
  line L657 (70.9952, 30.1924) -> (70.9952, 12.3524)
  line L658 (101.312, 69.307) -> (102.642, 69.307)
  line L659 (101.312, 67.977) -> (101.312, 69.307)
  line L660 (101.312, 66.707) -> (101.312, 48.867)
  line L661 (101.312, 66.707) -> (103.972, 66.707)
  line L662 (101.312, 48.867) -> (103.972, 48.867)
  line L663 (103.972, 66.707) -> (103.972, 48.867)
  line L664 (29.9816, 0.6574) -> (28.6516, 0.6574)
  line L665 (29.9816, 1.9874) -> (29.9816, 0.6574)
  line L666 (29.9816, 3.2574) -> (29.9816, 21.0974)
  line L667 (29.9816, 3.2574) -> (27.3216, 3.2574)
  line L668 (29.9816, 21.0974) -> (27.3216, 21.0974)
  line L669 (27.3216, 3.2574) -> (27.3216, 21.0974)
  line L670 (129.81, 0.6866) -> (128.48, 0.6866)
  line L671 (129.81, 2.0166) -> (129.81, 0.6866)
  line L672 (129.81, 3.2866) -> (129.81, 21.1266)
  line L673 (129.81, 3.2866) -> (127.15, 3.2866)
  line L674 (129.81, 21.1266) -> (127.15, 21.1266)
  line L675 (127.15, 3.2866) -> (127.15, 21.1266)
  line L676 (1.5836, 32.7778) -> (2.9136, 32.7778)
  line L677 (1.5836, 31.4478) -> (1.5836, 32.7778)
  line L678 (1.5836, 30.1778) -> (1.5836, 12.3378)
  line L679 (1.5836, 30.1778) -> (4.2436, 30.1778)
  line L680 (1.5836, 12.3378) -> (4.2436, 12.3378)
  line L681 (4.2436, 30.1778) -> (4.2436, 12.3378)
  line L682 (62.9582, 37.172) -> (61.6282, 37.172)
  line L683 (62.9582, 38.502) -> (62.9582, 37.172)
  line L684 (62.9582, 39.772) -> (62.9582, 57.612)
  line L685 (62.9582, 39.772) -> (60.2982, 39.772)
  line L686 (62.9582, 57.612) -> (60.2982, 57.612)
  line L687 (60.2982, 39.772) -> (60.2982, 57.612)
  line L688 (96.7332, 0.672) -> (95.4032, 0.672)
  line L689 (96.7332, 2.002) -> (96.7332, 0.672)
  line L690 (96.7332, 3.272) -> (96.7332, 21.112)
  line L691 (96.7332, 3.272) -> (94.0732, 3.272)
  line L692 (96.7332, 21.112) -> (94.0732, 21.112)
  line L693 (94.0732, 3.272) -> (94.0732, 21.112)
  line L694 (68.2352, 69.2924) -> (69.5652, 69.2924)
  line L695 (68.2352, 67.9624) -> (68.2352, 69.2924)
  line L696 (68.2352, 66.6924) -> (68.2352, 48.8524)
  line L697 (68.2352, 66.6924) -> (70.8952, 66.6924)
  line L698 (68.2352, 48.8524) -> (70.8952, 48.8524)
  line L699 (70.8952, 66.6924) -> (70.8952, 48.8524)
  line L700 (1.4836, 69.2778) -> (2.8136, 69.2778)
  line L701 (1.4836, 67.9478) -> (1.4836, 69.2778)
  line L702 (1.4836, 66.6778) -> (1.4836, 48.8378)
  line L703 (1.4836, 66.6778) -> (4.1436, 66.6778)
  line L704 (1.4836, 48.8378) -> (4.1436, 48.8378)
  line L705 (4.1436, 66.6778) -> (4.1436, 48.8378)
  line L706 (29.8816, 37.1574) -> (28.5516, 37.1574)
  line L707 (29.8816, 38.4874) -> (29.8816, 37.1574)
  line L708 (29.8816, 39.7574) -> (29.8816, 57.5974)
  line L709 (29.8816, 39.7574) -> (27.2216, 39.7574)
  line L710 (29.8816, 57.5974) -> (27.2216, 57.5974)
  line L711 (27.2216, 39.7574) -> (27.2216, 57.5974)
  line L712 (34.6602, 32.7924) -> (35.9902, 32.7924)
  line L713 (34.6602, 31.4624) -> (34.6602, 32.7924)
  line L714 (34.6602, 30.1924) -> (34.6602, 12.3524)
  line L715 (34.6602, 30.1924) -> (37.3202, 30.1924)
  line L716 (34.6602, 12.3524) -> (37.3202, 12.3524)
  line L717 (37.3202, 30.1924) -> (37.3202, 12.3524)
  line L718 (101.412, 32.807) -> (102.742, 32.807)
  line L719 (101.412, 31.477) -> (101.412, 32.807)
  line L720 (101.412, 30.207) -> (101.412, 12.367)
  line L721 (101.412, 30.207) -> (104.072, 30.207)
  line L722 (101.412, 12.367) -> (104.072, 12.367)
  line L723 (104.072, 30.207) -> (104.072, 12.367)
  line L724 (129.71, 37.1866) -> (128.38, 37.1866)
  line L725 (129.71, 38.5166) -> (129.71, 37.1866)
  line L726 (129.71, 39.7866) -> (129.71, 57.6266)
  line L727 (129.71, 39.7866) -> (127.05, 39.7866)
  line L728 (129.71, 57.6266) -> (127.05, 57.6266)
  line L729 (127.05, 39.7866) -> (127.05, 57.6266)
  line L730 (63.0582, 0.672) -> (61.7282, 0.672)
  line L731 (63.0582, 2.002) -> (63.0582, 0.672)
  line L732 (63.0582, 3.272) -> (63.0582, 21.112)
  line L733 (63.0582, 3.272) -> (60.3982, 3.272)
  line L734 (63.0582, 21.112) -> (60.3982, 21.112)
  line L735 (60.3982, 3.272) -> (60.3982, 21.112)
  line L736 (-2.525, 73.7982) -> (137.2, 73.7982)
  line L737 (137.2, 73.7982) -> (137.2, -4.8272)
  line L738 (137.2, -4.8272) -> (-2.525, -4.8272)
  line L739 (-2.525, -4.8272) -> (-2.525, 73.7982)
  point P0 (0, 0)
  point P1 (29.62197, 0.0124)
  point P2 (29.68123, 0.0124)
  point P3 (30.38387, 0.0124)
  point P4 (30.44313, 0.0124)
  point P5 (26.7468, 0.0124)
  point P6 (26.7468, 0.29)
  point P7 (27.3183, 0.0124)
  point P8 (0.125, 33.4228)
  point P9 (29.52197, 36.5124)
  point P10 (29.58123, 36.5124)
  point P11 (30.28387, 36.5124)
  point P12 (30.34313, 36.5124)
  point P13 (1.4266, 47.4594)
  point P14 (26.6468, 36.5124)
  point P15 (27.2183, 36.5124)
  point P16 (0.025, 69.9228)
  point P17 (62.59857, 36.527)
  point P18 (62.65783, 36.527)
  point P19 (63.36047, 36.527)
  point P20 (63.41973, 36.527)
  point P21 (59.7234, 36.527)
  point P22 (60.2949, 36.527)
  point P23 (62.69857, 0.027)
  point P24 (62.75783, 0.027)
  point P25 (63.46047, 0.027)
  point P26 (63.51973, 0.027)
  point P27 (42.8532, 0.027)
  point P28 (59.8234, 0.027)
  point P29 (60.3949, 0.027)
  point P30 (96.37357, 0.027)
  point P31 (96.43283, 0.027)
  point P32 (97.13547, 0.027)
  point P33 (97.19473, 0.027)
  point P34 (93.4984, 0.027)
  point P35 (94.0699, 0.027)
  point P36 (96.27357, 36.527)
  point P37 (96.33283, 36.527)
  point P38 (97.03547, 36.527)
  point P39 (97.09473, 36.527)
  point P40 (93.3984, 36.527)
  point P41 (93.9699, 36.527)
  point P42 (129.350349, 36.5416)
  point P43 (129.409651, 36.5416)
  point P44 (130.112349, 36.5416)
  point P45 (130.171651, 36.5416)
  point P46 (126.475, 36.5416)
  point P47 (127.046, 36.5416)
  point P48 (129.450349, 0.0416)
  point P49 (129.509651, 0.0416)
  point P50 (130.212349, 0.0416)
  point P51 (130.271651, 0.0416)
  point P52 (126.575, 0.0416)
  point P53 (127.147, 0.0416)
  constraints: 1480 end point